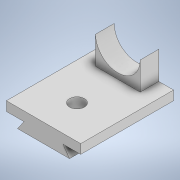
# Autodesk Inventor part: 2-6
Saved by Autodesk Inventor 2020 (Build 240168000, 168)
## iProperties
Created: 2023-12-07
Part Number: 2-6
Material: 常规
Document SubType Name: Modeling
Designer: Z
Density: 1 g/cm^3
Appearance: 默认
Author: Z
Autodesk Inventor part; units mm, degrees
ref_plane "YZ Plane" through (0, 0, 0) normal (1, 0, 0) x (0, 1, 0)
ref_plane "XZ Plane" through (0, 0, 0) normal (0, 1, 0) x (-1, 0, 0)
ref_plane "XY Plane" through (0, 0, 0) normal (0, 0, 1) x (1, 0, 0)
sketch "草图1" plane through (0, 0, 0) normal (0, 0, 1) x (1, 0, 0)
  line L0 (0, 0) -> (0, 17.5565)
  line L1 (-20, 2.5) -> (20, 2.5)
  line L2 (20, 2.5) -> (20, -2.5)
  line L3 (-20, -2.5) -> (-20, 2.5)
  line L4 (-20, 2.5) -> (20, -2.5) construction
  line L5 (20, 2.5) -> (-20, -2.5) construction
  line L6 (0, -7.5) -> (14, -7.5)
  line L7 (0, -7.5) -> (-14, -7.5)
  line L8 (-10.5, -2.5) -> (-14, -7.5)
  line L9 (14, -7.5) -> (10.5, -2.5)
  line L10 (20, -2.5) -> (10.5, -2.5)
  line L11 (-10.5, -2.5) -> (-20, -2.5)
  dimension "d1" = 40
  dimension "d2" = 5
  dimension "d5" = 14
  dimension "d8" = 21
  constraints: 24 end point, 3 horizontal, 3 parallel, 2 midpoint, 1 perpendicular, 1 vertical
  measures "d1" distance of L2.end L3.start
  measures "d2" distance of L1.end L2.end
  measures "d5" distance of L6.start L7.end
  measures "d8" distance of L9.end L8.start
extrude "拉伸1" add sketch "草图1" along normal blind 50
sketch "草图2" plane through (0, 0, 0) normal (0, 0, -1) x (-1, 0, 0)
  line L0 (-20, 2.5) -> (20, 2.5) projected
  line L1 (0, 2.5) -> (0, 17.5)
  arc A0 (-12, 17.5) -> (12, 17.5) centre (0, 17.5) ccw
  line L2 (-12, 17.5) -> (-12, 2.5)
  line L3 (12, 17.5) -> (12, 2.5)
  point P0 (0, 0)
  dimension "d11" = 15
  dimension "d12" = 24
  constraints: 6 end point, 2 perpendicular, 2 point on circle, 2 point on line, 2 tangent, 1 centre point, 1 coincident, 1 midpoint, 1 vertical
  measures "d11" distance of L1.start L1.end
  measures "d12" diameter of A0
extrude "拉伸2" add sketch "草图2" against normal blind 10
sketch "草图3" plane through (-20, 2.5, 50) normal (0, 1, 0) x (1, 0, 0)
  line L0 (40, 0) -> (0, 0) projected
  line L1 (20, 0) -> (20, 18)
  circle A0 centre (20, 18) radius 4
  point P0 (20, 50)
  dimension "d15" = 18
  dimension "d16" = 8
  constraints: 2 end point, 1 centre point, 1 coincident, 1 midpoint, 1 vertical
  measures "d15" distance of L1.start L1.end
  measures "d16" diameter of A0
extrude "拉伸3" cut sketch "草图3" against normal blind 20
